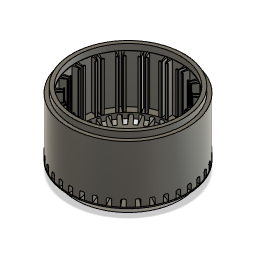
Halbach_Rotor_A (Autodesk Fusion 360 design; units mm, degrees)
Autodesk Fusion 360 part; units mm, degrees
note: some values were not read from the file. Chosen so that the rebuilt part matches the saved one: which face or edge a step refers to.
(part 1 of 3)
sketch "Sketch1" plane through (0, 0, 0) normal (0, 1, 0) x (1, 0, 0)
  line L0 (-5.9762, 42.5827) -> (4.023, 42.711)
  line L1 (-6.5833, 37.3358) -> (-7.4669, 42.3467) construction
  line L2 (-7.4669, 42.3467) -> (-6.3685, 36.1175)
  line L3 (0, 0) -> (7.4669, 42.3467) construction
  arc A0 (-6.7723, 38.4075) -> (-19.5, 33.775) centre (0, 0) ccw construction
  arc A1 (7.4669, 42.3467) -> (-7.4669, 42.3467) centre (0, 0) ccw construction
  line L4 (0, 0) -> (0, 22.1524)
  line L5 (5.4237, 42.6398) -> (7.4669, 42.3467)
  line L6 (4.023, 42.711) -> (4.0904, 37.4578)
  arc A2 (19.5, 33.775) -> (6.7723, 38.4075) centre (0, 0) ccw construction
  line L7 (-7.4669, 42.3467) -> (-5.9762, 42.5827)
  line L8 (-5.9762, 42.5827) -> (-5.912, 37.5831)
  line L9 (5.4238, 42.6403) -> (4.6599, 37.3153)
  line L10 (-5.912, 37.5831) -> (-5.9313, 39.0855)
  line L11 (7.4669, 42.3467) -> (6.4589, 36.6302)
  arc A3 (21.4323, 37.2711) -> (7.4669, 42.3467) centre (0.1099, 0.3541) ccw construction
  arc A4 (-7.2932, 41.3619) -> (-21, 36.3731) centre (0, 0) ccw construction
  line L12 (-5.912, 37.5831) -> (-4.4122, 37.6023)
  line L13 (-4.4122, 37.6023) -> (-4.4057, 37.1024)
  line L14 (-4.4057, 37.1024) -> (-5.9663, 36.8865)
  line L15 (4.0904, 37.4578) -> (2.5905, 37.4386)
  line L16 (2.5905, 37.4386) -> (2.5969, 36.9386)
  line L17 (4.6169, 36.9835) -> (4.6139, 36.9628)
  line L18 (-7.4669, 42.3467) -> (-6.4589, 36.6302)
  line L19 (-9.4242, 41.9378) -> (-7.4669, 42.3467)
  arc A5 (-7.4669, 42.3467) -> (-21.5, 37.2391) centre (0, 0) ccw construction
  line L20 (-23.1994, 36.1854) -> (-21.5, 37.2391)
  arc A6 (-21.5, 37.2391) -> (-32.9399, 27.6399) centre (0, 0) ccw construction
  line L21 (-34.1765, 26.0685) -> (-32.9399, 27.6399)
  arc A7 (-32.9399, 27.6399) -> (-40.4068, 14.7069) centre (0, 0) ccw construction
  line L22 (-41.0313, 12.8073) -> (-40.4068, 14.7069)
  arc A8 (-40.4068, 14.7069) -> (-43, 0) centre (0, 0) ccw construction
  line L23 (-42.9372, -1.9986) -> (-43, 0)
  arc A9 (-43, 0) -> (-40.4068, -14.7069) centre (0, 0) ccw construction
  line L24 (-39.6642, -16.5635) -> (-40.4068, -14.7069)
  arc A10 (-40.4068, -14.7069) -> (-32.9399, -27.6399) centre (0, 0) ccw construction
  line L25 (-31.6071, -29.1305) -> (-32.9399, -27.6399)
  arc A11 (-32.9399, -27.6399) -> (-21.5, -37.2391) centre (0, 0) ccw construction
  line L26 (-19.7377, -38.184) -> (-21.5, -37.2391)
  arc A12 (-21.5, -37.2391) -> (-7.4669, -42.3467) centre (0, 0) ccw construction
  line L27 (-5.4877, -42.6319) -> (-7.4669, -42.3467)
  arc A13 (-7.4669, -42.3467) -> (7.4669, -42.3467) centre (0, 0) ccw construction
  line L28 (21.5, -37.2391) -> (20.1799, -37.9707)
  line L29 (21.5, -37.2391) -> (18.3374, -31.7612)
  line L30 (9.4242, -41.9378) -> (7.4669, -42.3467)
  arc A14 (7.4669, -42.3467) -> (21.5, -37.2391) centre (0, 0) ccw construction
  line L31 (21.5, -37.2391) -> (18.5976, -32.212)
  line L32 (23.1994, -36.1854) -> (21.5, -37.2391)
  arc A15 (21.5, -37.2391) -> (32.9399, -27.6399) centre (0, 0) ccw construction
  line L33 (34.1765, -26.0685) -> (32.9399, -27.6399)
  arc A16 (32.9399, -27.6399) -> (40.4068, -14.7069) centre (0, 0) ccw construction
  line L34 (41.0313, -12.8073) -> (40.4068, -14.7069)
  arc A17 (40.4068, -14.7069) -> (43, 0) centre (0, 0) ccw construction
  line L35 (42.9372, 1.9986) -> (43, 0)
  arc A18 (43, 0) -> (40.4068, 14.7069) centre (0, 0) ccw construction
  line L36 (39.6642, 16.5635) -> (40.4068, 14.7069)
  arc A19 (40.4068, 14.7069) -> (32.9399, 27.6399) centre (0, 0) ccw construction
  line L37 (31.6071, 29.1305) -> (32.9399, 27.6399)
  arc A20 (32.9399, 27.6399) -> (21.5, 37.2391) centre (0, 0) ccw construction
  line L38 (19.7377, 38.184) -> (21.5, 37.2391)
  arc A21 (21.5, 37.2391) -> (7.4669, 42.3467) centre (0, 0) ccw construction
  line L39 (-9.4242, 41.9378) -> (-9.4276, 41.9538)
  arc A22 (-6.5833, 37.3358) -> (-5.9663, 36.8865) centre (-6.0417, 37.4314) ccw
  line L40 (4.73, 37.8039) -> (4.6599, 37.3153)
  line L41 (4.1482, 36.8865) -> (2.5969, 36.9386)
  arc A23 (4.1482, 36.8865) -> (4.6599, 37.3153) centre (4.165, 37.3863) ccw
  line L42 (-18.9559, 32.8326) -> (-21.5, 37.2391) construction
  line L43 (-9.4871, 41.9233) -> (-7.4669, 42.3467)
  line L44 (-8.3107, 36.3322) -> (-8.3064, 36.3118)
  line L45 (-10.8276, 41.5111) -> (-8.9676, 36.5978)
  line L46 (-7.4669, 42.3467) -> (-6.4589, 36.6302)
  line L47 (-9.4872, 41.9238) -> (-8.3837, 36.6587)
  line L48 (-23.1994, 36.1854) -> (-23.208, 36.1993)
  line L49 (-8.4849, 37.1418) -> (-8.3837, 36.6587)
  line L50 (-8.9676, 36.5978) -> (-10.3705, 36.0667)
  line L51 (-20.1799, 37.9707) -> (-18.4097, 33.2945)
  line L52 (-10.3705, 36.0667) -> (-10.1934, 35.5991)
  line L53 (-8.7179, 36.0808) -> (-10.1934, 35.5991)
  line L54 (-16.8298, 33.358) -> (-18.2224, 32.6214)
  line L55 (-21.5, 37.2391) -> (-18.5976, 32.212)
  line L56 (-23.1994, 36.1854) -> (-21.5, 37.2391)
  arc A24 (-7.4669, 42.3467) -> (-21.5, 37.2391) centre (0, 0) ccw construction
  line L57 (-20.1799, 37.9707) -> (-10.8276, 41.5111)
  line L58 (-21.5, 37.2391) -> (-20.1799, 37.9707)
  arc A25 (-18.9559, 32.8326) -> (-18.2224, 32.6214) centre (-18.4796, 33.1076) ccw
  line L59 (-18.4097, 33.2945) -> (-18.9416, 34.6997)
  line L60 (-18.4097, 33.2945) -> (-17.0068, 33.8256)
  line L61 (-17.0068, 33.8256) -> (-16.8298, 33.358)
  line L62 (-21.5, 37.2391) -> (-18.3374, 31.7612)
  arc A26 (-8.7179, 36.0808) -> (-8.3837, 36.6587) centre (-8.873, 36.5561) ccw
  line L63 (-29.0421, 24.3692) -> (-32.9399, 27.6399) construction
  line L64 (-23.2536, 36.1503) -> (-21.5, 37.2391)
  line L65 (-20.2358, 31.2987) -> (-20.2248, 31.2809)
  line L66 (-24.3723, 35.3044) -> (-20.944, 31.3236)
  line L67 (-21.5, 37.2391) -> (-18.5976, 32.212)
  line L68 (-23.2538, 36.1507) -> (-20.4161, 31.5805)
  line L69 (-34.1765, 26.0685) -> (-34.1893, 26.0786)
  line L70 (-20.6765, 31.9999) -> (-20.4161, 31.5805)
  line L71 (-20.944, 31.3236) -> (-22.0806, 30.3448)
  line L72 (-31.9496, 28.7788) -> (-28.6868, 24.9901)
  line L73 (-22.0806, 30.3448) -> (-21.7543, 29.9659)
  line L74 (-20.5325, 30.9232) -> (-21.7543, 29.9659)
  line L75 (-27.2239, 25.5901) -> (-28.2807, 24.4217)
  line L76 (-32.9399, 27.6399) -> (-28.4932, 23.9087)
  line L77 (-34.1765, 26.0685) -> (-32.9399, 27.6399)
  arc A27 (-21.5, 37.2391) -> (-32.9399, 27.6399) centre (0, 0) ccw construction
  line L78 (-31.9496, 28.7788) -> (-24.3723, 35.3044)
  line L79 (-32.9399, 27.6399) -> (-31.9496, 28.7788)
  arc A28 (-29.0421, 24.3692) -> (-28.2807, 24.4217) centre (-28.6886, 24.7906) ccw
  line L80 (-28.6868, 24.9901) -> (-29.6673, 26.1287)
  line L81 (-28.6868, 24.9901) -> (-27.5502, 25.969)
  line L82 (-27.5502, 25.969) -> (-27.2239, 25.5901)
  line L83 (-32.9399, 27.6399) -> (-28.0945, 23.5741)
  arc A29 (-20.5325, 30.9232) -> (-20.4161, 31.5805) centre (-20.8408, 31.3168) ccw
  line L84 (-35.6255, 12.9666) -> (-40.4068, 14.7069) construction
  line L85 (-34.2153, 26.0169) -> (-32.9399, 27.6399)
  line L86 (-29.7202, 22.4901) -> (-29.7038, 22.4772)
  line L87 (-34.9773, 24.8395) -> (-30.3942, 22.2713)
  line L88 (-32.9399, 27.6399) -> (-28.4932, 23.9087)
  line L89 (-34.2157, 26.0173) -> (-29.986, 22.6933)
  line L90 (-41.0313, 12.8073) -> (-41.0468, 12.8124)
  line L91 (-30.3741, 22.9983) -> (-29.986, 22.6933)
  line L92 (-30.3942, 22.2713) -> (-31.1275, 20.9627)
  line L93 (-39.8658, 16.1158) -> (-35.5039, 13.6716)
  line L94 (-31.1275, 20.9627) -> (-30.6913, 20.7183)
  line L95 (-29.8706, 22.0358) -> (-30.6913, 20.7183)
  line L96 (-34.3345, 14.7357) -> (-34.9278, 13.2763)
  line L97 (-40.4068, 14.7069) -> (-34.9521, 12.7215)
  line L98 (-41.0313, 12.8073) -> (-40.4068, 14.7069)
  arc A30 (-32.9399, 27.6399) -> (-40.4068, 14.7069) centre (0, 0) ccw construction
  line L99 (-39.8658, 16.1158) -> (-34.9773, 24.8395)
  line L100 (-40.4068, 14.7069) -> (-39.8658, 16.1158)
  arc A31 (-35.6255, 12.9666) -> (-34.9278, 13.2763) centre (-35.4373, 13.4834) ccw
  line L101 (-35.5039, 13.6716) -> (-36.8147, 14.4061)
  line L102 (-35.5039, 13.6716) -> (-34.7707, 14.9801)
  line L103 (-34.7707, 14.9801) -> (-34.3345, 14.7357)
  line L104 (-40.4068, 14.7069) -> (-34.463, 12.5435)
  arc A32 (-29.8706, 22.0358) -> (-29.986, 22.6933) centre (-30.2949, 22.3001) ccw
  line L105 (-37.9118, 0) -> (-43, 0) construction
  line L106 (-41.0502, 12.7456) -> (-40.4068, 14.7069)
  line L107 (-35.6199, 10.9688) -> (-35.6001, 10.9623)
  line L108 (-41.3635, 11.3786) -> (-36.1784, 10.5327)
  line L109 (-40.4068, 14.7069) -> (-34.9521, 12.7215)
  line L110 (-41.0507, 12.7458) -> (-35.9392, 11.0689)
  line L111 (-42.9372, -1.9986) -> (-42.9535, -1.9991)
  line L112 (-36.4082, 11.2228) -> (-35.9392, 11.0689)
  line L113 (-36.1784, 10.5327) -> (-36.4199, 9.0523)
  line L114 (-42.9735, 1.509) -> (-38.0387, 0.704)
  line L115 (-36.4199, 9.0523) -> (-35.9265, 8.9718)
  line L116 (-35.6058, 10.4905) -> (-35.9265, 8.9718)
  line L117 (-37.3038, 2.1039) -> (-37.3622, 0.5296)
  line L118 (-43, 0) -> (-37.1953, 0)
  line L119 (-42.9372, -1.9986) -> (-43, 0)
  arc A33 (-40.4068, 14.7069) -> (-43, 0) centre (0, 0) ccw construction
  line L120 (-42.9735, 1.509) -> (-41.3635, 11.3786)
  line L121 (-43, 0) -> (-42.9735, 1.509)
  arc A34 (-37.9118, 0) -> (-37.3622, 0.5296) centre (-37.9118, 0.55) ccw
  line L122 (-38.0387, 0.704) -> (-39.5217, 0.9459)
  line L123 (-38.0387, 0.704) -> (-37.7972, 2.1844)
  line L124 (-37.7972, 2.1844) -> (-37.3038, 2.1039)
  line L125 (-43, 0) -> (-36.6747, 0)
  arc A35 (-35.6058, 10.4905) -> (-35.9392, 11.0689) centre (-36.095, 10.5938) ccw
  line L126 (-35.6255, -12.9666) -> (-40.4068, -14.7069) construction
  line L127 (-42.9338, -2.063) -> (-43, 0)
  line L128 (-37.2233, -1.8754) -> (-37.2025, -1.8747)
  line L129 (-42.7607, -3.4548) -> (-37.599, -2.4762)
  line L130 (-43, 0) -> (-37.1953, 0)
  line L131 (-42.9343, -2.0631) -> (-37.5576, -1.8906)
  line L132 (-39.6642, -16.5635) -> (-39.6793, -16.5695)
  line L133 (-38.0509, -1.9064) -> (-37.5576, -1.8906)
  line L134 (-37.599, -2.4762) -> (-37.3196, -3.95)
  line L135 (-40.898, -13.2798) -> (-35.9855, -12.3485)
  line L136 (-37.3196, -3.95) -> (-36.8284, -3.8568)
  line L137 (-37.0465, -2.3201) -> (-36.8284, -3.8568)
  line L138 (-35.7737, -10.7816) -> (-35.2901, -12.281)
  line L139 (-40.4068, -14.7069) -> (-34.9521, -12.7215)
  line L140 (-39.6642, -16.5635) -> (-40.4068, -14.7069)
  arc A36 (-43, 0) -> (-40.4068, -14.7069) centre (0, 0) ccw construction
  line L141 (-40.898, -13.2798) -> (-42.7607, -3.4548)
  line L142 (-40.4068, -14.7069) -> (-40.898, -13.2798)
  arc A37 (-35.6255, -12.9666) -> (-35.2901, -12.281) centre (-35.8136, -12.4498) ccw
  line L143 (-35.9855, -12.3485) -> (-37.4617, -12.6283)
  line L144 (-35.9855, -12.3485) -> (-36.2649, -10.8747)
  line L145 (-36.2649, -10.8747) -> (-35.7737, -10.7816)
  line L146 (-40.4068, -14.7069) -> (-34.463, -12.5435)
  arc A38 (-37.0465, -2.3201) -> (-37.5576, -1.8906) centre (-37.5415, -2.3903) ccw
  line L147 (-29.0421, -24.3692) -> (-32.9399, -27.6399) construction
  line L148 (-39.639, -16.6229) -> (-40.4068, -14.7069)
  line L149 (-34.3371, -14.4934) -> (-34.3177, -14.4857)
  line L150 (-39.0003, -17.8714) -> (-34.4846, -15.1865)
  line L151 (-40.4068, -14.7069) -> (-34.9521, -12.7215)
  line L152 (-39.6395, -16.623) -> (-34.6459, -14.622)
  line L153 (-31.6071, -29.1305) -> (-31.6193, -29.1414)
  line L154 (-35.1041, -14.8056) -> (-34.6459, -14.622)
  line L155 (-34.4846, -15.1865) -> (-33.718, -16.4758)
  line L156 (-33.8896, -26.4669) -> (-29.5919, -23.9115)
  line L157 (-33.718, -16.4758) -> (-33.2882, -16.2203)
  line L158 (-34.0188, -14.8508) -> (-33.2882, -16.2203)
  line L159 (-29.9287, -22.3667) -> (-28.9615, -23.6103)
  line L160 (-32.9399, -27.6399) -> (-28.4932, -23.9087)
  line L161 (-31.6071, -29.1305) -> (-32.9399, -27.6399)
  arc A39 (-40.4068, -14.7069) -> (-32.9399, -27.6399) centre (0, 0) ccw construction
  line L162 (-33.8896, -26.4669) -> (-39.0003, -17.8714)
  line L163 (-32.9399, -27.6399) -> (-33.8896, -26.4669)
  arc A40 (-29.0421, -24.3692) -> (-28.9615, -23.6103) centre (-29.3957, -23.9479) ccw
  line L164 (-29.5919, -23.9115) -> (-30.8834, -24.6794)
  line L165 (-29.5919, -23.9115) -> (-30.3585, -22.6222)
  line L166 (-30.3585, -22.6222) -> (-29.9287, -22.3667)
  line L167 (-32.9399, -27.6399) -> (-28.0945, -23.5741)
  arc A41 (-34.0188, -14.8508) -> (-34.6459, -14.622) centre (-34.46, -15.0861) ccw
  line L168 (-18.9559, -32.8326) -> (-21.5, -37.2391) construction
  line L169 (-31.5631, -29.1777) -> (-32.9399, -27.6399)
  line L170 (-27.3092, -25.3633) -> (-27.2937, -25.3494)
  line L171 (-30.5359, -30.1325) -> (-27.2108, -26.0651)
  line L172 (-32.9399, -27.6399) -> (-28.4932, -23.9087)
  line L173 (-31.5635, -29.178) -> (-27.5555, -25.5898)
  line L174 (-19.7377, -38.184) -> (-19.7455, -38.1984)
  line L175 (-27.9233, -25.9191) -> (-27.5555, -25.5898)
  line L176 (-27.2108, -26.0651) -> (-26.0495, -27.0145)
  line L177 (-22.7936, -36.4616) -> (-19.6291, -32.5905)
  line L178 (-26.0495, -27.0145) -> (-25.733, -26.6273)
  line L179 (-26.888, -25.5903) -> (-25.733, -26.6273)
  line L180 (-20.474, -31.254) -> (-19.1397, -32.0918)
  line L181 (-21.5, -37.2391) -> (-18.5976, -32.212)
  line L182 (-19.7377, -38.184) -> (-21.5, -37.2391)
  arc A42 (-32.9399, -27.6399) -> (-21.5, -37.2391) centre (0, 0) ccw construction
  line L183 (-22.7936, -36.4616) -> (-30.5359, -30.1325)
  line L184 (-21.5, -37.2391) -> (-22.7936, -36.4616)
  arc A43 (-18.9559, -32.8326) -> (-19.1397, -32.0918) centre (-19.4322, -32.5576) ccw
  line L185 (-19.6291, -32.5905) -> (-20.58, -33.7538)
  line L186 (-19.6291, -32.5905) -> (-20.7904, -31.6411)
  line L187 (-20.7904, -31.6411) -> (-20.474, -31.254)
  line L188 (-21.5, -37.2391) -> (-18.3374, -31.7612)
  arc A44 (-26.888, -25.5903) -> (-27.5555, -25.5898) centre (-27.222, -25.9623) ccw
  line L189 (-6.5833, -37.3358) -> (-7.4669, -42.3467) construction
  line L190 (-19.6803, -38.2133) -> (-21.5, -37.2391)
  line L191 (-16.9875, -33.1741) -> (-16.9777, -33.1557)
  line L192 (-18.3884, -38.7592) -> (-16.655, -33.7998)
  line L193 (-21.5, -37.2391) -> (-18.5976, -32.212)
  line L194 (-19.6805, -38.2137) -> (-17.1415, -33.4711)
  line L195 (-5.4877, -42.6319) -> (-5.49, -42.6481)
  line L196 (-17.3745, -33.9063) -> (-17.1415, -33.4711)
  line L197 (-16.655, -33.7998) -> (-15.239, -34.2947)
  line L198 (-8.9484, -42.0586) -> (-7.2987, -37.3386)
  line L199 (-15.239, -34.2947) -> (-15.0741, -33.8227)
  line L200 (-16.514, -33.2432) -> (-15.0741, -33.8227)
  line L201 (-8.5497, -36.3717) -> (-7.0094, -36.7026)
  line L202 (-7.4669, -42.3467) -> (-6.4589, -36.6302)
  line L203 (-5.4877, -42.6319) -> (-7.4669, -42.3467)
  arc A45 (-21.5, -37.2391) -> (-7.4669, -42.3467) centre (0, 0) ccw construction
  line L204 (-8.9484, -42.0586) -> (-18.3884, -38.7592)
  line L205 (-7.4669, -42.3467) -> (-8.9484, -42.0586)
  arc A46 (-6.5833, -37.3358) -> (-7.0094, -36.7026) centre (-7.125, -37.2403) ccw
  line L206 (-7.2987, -37.3386) -> (-7.7944, -38.757)
  line L207 (-7.2987, -37.3386) -> (-8.7147, -36.8437)
  line L208 (-8.7147, -36.8437) -> (-8.5497, -36.3717)
  line L209 (-7.4669, -42.3467) -> (-6.3685, -36.1175)
  arc A47 (-16.514, -33.2432) -> (-17.1415, -33.4711) centre (-16.7007, -33.7071) ccw
  line L210 (6.5833, -37.3358) -> (7.4669, -42.3467) construction
  line L211 (-5.4237, -42.6398) -> (-7.4669, -42.3467)
  line L212 (-4.6169, -36.9835) -> (-4.6139, -36.9628)
  line L213 (-4.023, -42.711) -> (-4.0904, -37.4578)
  line L214 (-7.4669, -42.3467) -> (-6.4589, -36.6302)
  line L215 (-5.4238, -42.6403) -> (-4.6599, -37.3153)
  line L216 (9.4242, -41.9378) -> (9.4276, -41.9538)
  line L217 (-4.73, -37.8039) -> (-4.6599, -37.3153)
  line L218 (-4.0904, -37.4578) -> (-2.5905, -37.4386)
  line L219 (5.9762, -42.5827) -> (5.912, -37.5831)
  line L220 (-2.5905, -37.4386) -> (-2.5969, -36.9386)
  line L221 (-4.1482, -36.8865) -> (-2.5969, -36.9386)
  line L222 (4.4057, -37.1024) -> (5.9663, -36.8865)
  line L223 (7.4669, -42.3467) -> (6.4589, -36.6302)
  line L224 (9.4242, -41.9378) -> (7.4669, -42.3467)
  arc A48 (-7.4669, -42.3467) -> (7.4669, -42.3467) centre (0, 0) ccw construction
  line L225 (5.9762, -42.5827) -> (-4.023, -42.711)
  line L226 (7.4669, -42.3467) -> (5.9762, -42.5827)
  arc A49 (6.5833, -37.3358) -> (5.9663, -36.8865) centre (6.0417, -37.4314) ccw
  line L227 (5.912, -37.5831) -> (5.9313, -39.0855)
  line L228 (5.912, -37.5831) -> (4.4122, -37.6023)
  line L229 (4.4122, -37.6023) -> (4.4057, -37.1024)
  line L230 (7.4669, -42.3467) -> (6.3685, -36.1175)
  arc A50 (-4.1482, -36.8865) -> (-4.6599, -37.3153) centre (-4.165, -37.3863) ccw
  line L231 (18.9559, -32.8326) -> (21.5, -37.2391) construction
  line L232 (9.4871, -41.9233) -> (7.4669, -42.3467)
  line L233 (8.3107, -36.3322) -> (8.3064, -36.3118)
  line L234 (10.8276, -41.5111) -> (8.9676, -36.5978)
  line L235 (7.4669, -42.3467) -> (6.4589, -36.6302)
  line L236 (9.4872, -41.9238) -> (8.3837, -36.6587)
  line L237 (23.1994, -36.1854) -> (23.208, -36.1993)
  line L238 (8.4849, -37.1418) -> (8.3837, -36.6587)
  line L239 (8.9676, -36.5978) -> (10.3705, -36.0667)
  line L240 (20.1799, -37.9707) -> (18.4097, -33.2945)
  line L241 (10.3705, -36.0667) -> (10.1934, -35.5991)
  line L242 (8.7179, -36.0808) -> (10.1934, -35.5991)
  line L243 (16.8298, -33.358) -> (18.2224, -32.6214)
  line L244 (21.5, -37.2391) -> (18.5976, -32.212)
  line L245 (23.1994, -36.1854) -> (21.5, -37.2391)
  arc A51 (7.4669, -42.3467) -> (21.5, -37.2391) centre (0, 0) ccw construction
  line L246 (20.1799, -37.9707) -> (10.8276, -41.5111)
  line L247 (21.5, -37.2391) -> (20.1799, -37.9707)
  arc A52 (18.9559, -32.8326) -> (18.2224, -32.6214) centre (18.4796, -33.1076) ccw
  line L248 (18.4097, -33.2945) -> (18.9416, -34.6997)
  line L249 (18.4097, -33.2945) -> (17.0068, -33.8256)
  line L250 (17.0068, -33.8256) -> (16.8298, -33.358)
  line L251 (21.5, -37.2391) -> (18.3374, -31.7612)
  arc A53 (8.7179, -36.0808) -> (8.3837, -36.6587) centre (8.873, -36.5561) ccw
  line L252 (29.0421, -24.3692) -> (32.9399, -27.6399) construction
  line L253 (23.2536, -36.1503) -> (21.5, -37.2391)
  line L254 (20.2358, -31.2987) -> (20.2248, -31.2809)
  line L255 (24.3723, -35.3044) -> (20.944, -31.3236)
  line L256 (21.5, -37.2391) -> (18.5976, -32.212)
  line L257 (23.2538, -36.1507) -> (20.4161, -31.5805)
  line L258 (34.1765, -26.0685) -> (34.1893, -26.0786)
  line L259 (20.6765, -31.9999) -> (20.4161, -31.5805)
  line L260 (20.944, -31.3236) -> (22.0806, -30.3448)
  line L261 (31.9496, -28.7788) -> (28.6868, -24.9901)
  line L262 (22.0806, -30.3448) -> (21.7543, -29.9659)
  line L263 (20.5325, -30.9232) -> (21.7543, -29.9659)
  line L264 (27.2239, -25.5901) -> (28.2807, -24.4217)
  line L265 (32.9399, -27.6399) -> (28.4932, -23.9087)
  line L266 (34.1765, -26.0685) -> (32.9399, -27.6399)
  arc A54 (21.5, -37.2391) -> (32.9399, -27.6399) centre (0, 0) ccw construction
  line L267 (31.9496, -28.7788) -> (24.3723, -35.3044)
  line L268 (32.9399, -27.6399) -> (31.9496, -28.7788)
  arc A55 (29.0421, -24.3692) -> (28.2807, -24.4217) centre (28.6886, -24.7906) ccw
  line L269 (28.6868, -24.9901) -> (29.6673, -26.1287)
  line L270 (28.6868, -24.9901) -> (27.5502, -25.969)
  line L271 (27.5502, -25.969) -> (27.2239, -25.5901)
  line L272 (32.9399, -27.6399) -> (28.0945, -23.5741)
  arc A56 (20.5325, -30.9232) -> (20.4161, -31.5805) centre (20.8408, -31.3168) ccw
  line L273 (35.6255, -12.9666) -> (40.4068, -14.7069) construction
  line L274 (34.2153, -26.0169) -> (32.9399, -27.6399)
  line L275 (29.7202, -22.4901) -> (29.7038, -22.4772)
  line L276 (34.9773, -24.8395) -> (30.3942, -22.2713)
  line L277 (32.9399, -27.6399) -> (28.4932, -23.9087)
  line L278 (34.2157, -26.0173) -> (29.986, -22.6933)
  line L279 (41.0313, -12.8073) -> (41.0468, -12.8124)
  line L280 (30.3741, -22.9983) -> (29.986, -22.6933)
  line L281 (30.3942, -22.2713) -> (31.1275, -20.9627)
  line L282 (39.8658, -16.1158) -> (35.5039, -13.6716)
  line L283 (31.1275, -20.9627) -> (30.6913, -20.7183)
  line L284 (29.8706, -22.0358) -> (30.6913, -20.7183)
  line L285 (34.3345, -14.7357) -> (34.9278, -13.2763)
  line L286 (40.4068, -14.7069) -> (34.9521, -12.7215)
  line L287 (41.0313, -12.8073) -> (40.4068, -14.7069)
  arc A57 (32.9399, -27.6399) -> (40.4068, -14.7069) centre (0, 0) ccw construction
  line L288 (39.8658, -16.1158) -> (34.9773, -24.8395)
  line L289 (40.4068, -14.7069) -> (39.8658, -16.1158)
  arc A58 (35.6255, -12.9666) -> (34.9278, -13.2763) centre (35.4373, -13.4834) ccw
  line L290 (35.5039, -13.6716) -> (36.8147, -14.4061)
  line L291 (35.5039, -13.6716) -> (34.7707, -14.9801)
  line L292 (34.7707, -14.9801) -> (34.3345, -14.7357)
  line L293 (40.4068, -14.7069) -> (34.463, -12.5435)
  arc A59 (29.8706, -22.0358) -> (29.986, -22.6933) centre (30.2949, -22.3001) ccw
  line L294 (37.9118, 0) -> (43, 0) construction
  line L295 (41.0502, -12.7456) -> (40.4068, -14.7069)
  line L296 (35.6199, -10.9688) -> (35.6001, -10.9623)
  line L297 (41.3635, -11.3786) -> (36.1784, -10.5327)
  line L298 (40.4068, -14.7069) -> (34.9521, -12.7215)
  line L299 (41.0507, -12.7458) -> (35.9392, -11.0689)
  line L300 (42.9372, 1.9986) -> (42.9535, 1.9991)
  line L301 (36.4082, -11.2228) -> (35.9392, -11.0689)
  line L302 (36.1784, -10.5327) -> (36.4199, -9.0523)
  line L303 (42.9735, -1.509) -> (38.0387, -0.704)
  line L304 (36.4199, -9.0523) -> (35.9265, -8.9718)
  line L305 (35.6058, -10.4905) -> (35.9265, -8.9718)
  line L306 (37.3038, -2.1039) -> (37.3622, -0.5296)
  line L307 (43, 0) -> (37.1953, 0)
  line L308 (42.9372, 1.9986) -> (43, 0)
  arc A60 (40.4068, -14.7069) -> (43, 0) centre (0, 0) ccw construction
  line L309 (42.9735, -1.509) -> (41.3635, -11.3786)
  line L310 (43, 0) -> (42.9735, -1.509)
  arc A61 (37.9118, 0) -> (37.3622, -0.5296) centre (37.9118, -0.55) ccw
  line L311 (38.0387, -0.704) -> (39.5217, -0.9459)
  line L312 (38.0387, -0.704) -> (37.7972, -2.1844)
  line L313 (37.7972, -2.1844) -> (37.3038, -2.1039)
  line L314 (43, 0) -> (36.6747, 0)
  arc A62 (35.6058, -10.4905) -> (35.9392, -11.0689) centre (36.095, -10.5938) ccw
  line L315 (35.6255, 12.9666) -> (40.4068, 14.7069) construction
  line L316 (42.9338, 2.063) -> (43, 0)
  line L317 (37.2233, 1.8754) -> (37.2025, 1.8747)
  line L318 (42.7607, 3.4548) -> (37.599, 2.4762)
  line L319 (43, 0) -> (37.1953, 0)
  line L320 (42.9343, 2.0631) -> (37.5576, 1.8906)
  line L321 (39.6642, 16.5635) -> (39.6793, 16.5695)
  line L322 (38.0509, 1.9064) -> (37.5576, 1.8906)
  line L323 (37.599, 2.4762) -> (37.3196, 3.95)
  line L324 (40.898, 13.2798) -> (35.9855, 12.3485)
  line L325 (37.3196, 3.95) -> (36.8284, 3.8568)
  line L326 (37.0465, 2.3201) -> (36.8284, 3.8568)
  line L327 (35.7737, 10.7816) -> (35.2901, 12.281)
  line L328 (40.4068, 14.7069) -> (34.9521, 12.7215)
  line L329 (39.6642, 16.5635) -> (40.4068, 14.7069)
  arc A63 (43, 0) -> (40.4068, 14.7069) centre (0, 0) ccw construction
  line L330 (40.898, 13.2798) -> (42.7607, 3.4548)
  line L331 (40.4068, 14.7069) -> (40.898, 13.2798)
  arc A64 (35.6255, 12.9666) -> (35.2901, 12.281) centre (35.8136, 12.4498) ccw
  line L332 (35.9855, 12.3485) -> (37.4617, 12.6283)
  line L333 (35.9855, 12.3485) -> (36.2649, 10.8747)
  line L334 (36.2649, 10.8747) -> (35.7737, 10.7816)
  line L335 (40.4068, 14.7069) -> (34.463, 12.5435)
  arc A65 (37.0465, 2.3201) -> (37.5576, 1.8906) centre (37.5415, 2.3903) ccw
  line L336 (29.0421, 24.3692) -> (32.9399, 27.6399) construction
  line L337 (39.639, 16.6229) -> (40.4068, 14.7069)
  line L338 (34.3371, 14.4934) -> (34.3177, 14.4857)
  line L339 (39.0003, 17.8714) -> (34.4846, 15.1865)
  line L340 (40.4068, 14.7069) -> (34.9521, 12.7215)
  line L341 (39.6395, 16.623) -> (34.6459, 14.622)
  line L342 (31.6071, 29.1305) -> (31.6193, 29.1414)
  line L343 (35.1041, 14.8056) -> (34.6459, 14.622)
  line L344 (34.4846, 15.1865) -> (33.718, 16.4758)
  line L345 (33.8896, 26.4669) -> (29.5919, 23.9115)
  line L346 (33.718, 16.4758) -> (33.2882, 16.2203)
  line L347 (34.0188, 14.8508) -> (33.2882, 16.2203)
  line L348 (29.9287, 22.3667) -> (28.9615, 23.6103)
  line L349 (32.9399, 27.6399) -> (28.4932, 23.9087)
  line L350 (31.6071, 29.1305) -> (32.9399, 27.6399)
  arc A66 (40.4068, 14.7069) -> (32.9399, 27.6399) centre (0, 0) ccw construction
  line L351 (33.8896, 26.4669) -> (39.0003, 17.8714)
  line L352 (32.9399, 27.6399) -> (33.8896, 26.4669)
  arc A67 (29.0421, 24.3692) -> (28.9615, 23.6103) centre (29.3957, 23.9479) ccw
  line L353 (29.5919, 23.9115) -> (30.8834, 24.6794)
  line L354 (29.5919, 23.9115) -> (30.3585, 22.6222)
  line L355 (30.3585, 22.6222) -> (29.9287, 22.3667)
  line L356 (32.9399, 27.6399) -> (28.0945, 23.5741)
  arc A68 (34.0188, 14.8508) -> (34.6459, 14.622) centre (34.46, 15.0861) ccw
  line L357 (18.9559, 32.8326) -> (21.5, 37.2391) construction
  line L358 (31.5631, 29.1777) -> (32.9399, 27.6399)
  line L359 (27.3092, 25.3633) -> (27.2937, 25.3494)
  line L360 (30.5359, 30.1325) -> (27.2108, 26.0651)
  line L361 (32.9399, 27.6399) -> (28.4932, 23.9087)
  line L362 (31.5635, 29.178) -> (27.5555, 25.5898)
  line L363 (19.7377, 38.184) -> (19.7455, 38.1984)
  line L364 (27.9233, 25.9191) -> (27.5555, 25.5898)
  line L365 (27.2108, 26.0651) -> (26.0495, 27.0145)
  line L366 (22.7936, 36.4616) -> (19.6291, 32.5905)
  line L367 (26.0495, 27.0145) -> (25.733, 26.6273)
  line L368 (26.888, 25.5903) -> (25.733, 26.6273)
  line L369 (20.474, 31.254) -> (19.1397, 32.0918)
  line L370 (21.5, 37.2391) -> (18.5976, 32.212)
  line L371 (19.7377, 38.184) -> (21.5, 37.2391)
  arc A69 (32.9399, 27.6399) -> (21.5, 37.2391) centre (0, 0) ccw construction
  line L372 (22.7936, 36.4616) -> (30.5359, 30.1325)
  line L373 (21.5, 37.2391) -> (22.7936, 36.4616)
  arc A70 (18.9559, 32.8326) -> (19.1397, 32.0918) centre (19.4322, 32.5576) ccw
  line L374 (19.6291, 32.5905) -> (20.58, 33.7538)
  line L375 (19.6291, 32.5905) -> (20.7904, 31.6411)
  line L376 (20.7904, 31.6411) -> (20.474, 31.254)
  line L377 (21.5, 37.2391) -> (18.3374, 31.7612)
  arc A71 (26.888, 25.5903) -> (27.5555, 25.5898) centre (27.222, 25.9623) ccw
  line L378 (6.5833, 37.3358) -> (7.4669, 42.3467) construction
  line L379 (19.6803, 38.2133) -> (21.5, 37.2391)
  line L380 (16.9875, 33.1741) -> (16.9777, 33.1557)
  line L381 (18.3884, 38.7592) -> (16.655, 33.7998)
  line L382 (21.5, 37.2391) -> (18.5976, 32.212)
  line L383 (19.6805, 38.2137) -> (17.1415, 33.4711)
  line L384 (5.4877, 42.6319) -> (5.49, 42.6481)
  line L385 (17.3745, 33.9063) -> (17.1415, 33.4711)
  line L386 (16.655, 33.7998) -> (15.239, 34.2947)
  line L387 (8.9484, 42.0586) -> (7.2987, 37.3386)
  line L388 (15.239, 34.2947) -> (15.0741, 33.8227)
  line L389 (16.514, 33.2432) -> (15.0741, 33.8227)
  line L390 (8.5497, 36.3717) -> (7.0094, 36.7026)
  line L391 (7.4669, 42.3467) -> (6.4589, 36.6302)
  line L392 (5.4877, 42.6319) -> (7.4669, 42.3467)
  arc A72 (21.5, 37.2391) -> (7.4669, 42.3467) centre (0, 0) ccw construction
  line L393 (8.9484, 42.0586) -> (18.3884, 38.7592)
  line L394 (7.4669, 42.3467) -> (8.9484, 42.0586)
  arc A73 (6.5833, 37.3358) -> (7.0094, 36.7026) centre (7.125, 37.2403) ccw
  line L395 (7.2987, 37.3386) -> (7.7944, 38.757)
  line L396 (7.2987, 37.3386) -> (8.7147, 36.8437)
  line L397 (8.7147, 36.8437) -> (8.5497, 36.3717)
  line L398 (7.4669, 42.3467) -> (6.3685, 36.1175)
  arc A74 (16.514, 33.2432) -> (17.1415, 33.4711) centre (16.7007, 33.7071) ccw
  circle A75 centre (0, 0) radius 49
  line L399 (-5.9663, 36.8865) -> (5.7522, 36.8865)
  point P0 (4.0904, 37.4578)
  point P1 (16.3645, 32.9385)
  point P2 (19.5, 33.775)
  point P3 (6.7723, 38.4075)
  point P4 (-8.6365, 35.7513)
  point P5 (-7.2932, 41.3619)
  point P6 (-6.7723, 38.4075)
  point P7 (-19.5, 33.775)
  point P8 (-19.5, 33.775)
  point P9 (-6.7723, 38.4075)
  point P10 (-8.9676, 36.5978)
  point P11 (-19.5, 33.775)
  point P12 (-21, 36.3731)
  point P13 (-21, 36.3731)
  point P14 (-20.3434, 30.6413)
  point P15 (-7.4669, 42.3467)
  point P16 (-6.7723, 38.4075)
  point P17 (-29.8757, 25.0687)
  point P18 (-19.5, 33.775)
  point P19 (-20.944, 31.3236)
  point P20 (-29.8757, 25.0687)
  point P21 (-32.1739, 26.9971)
  point P22 (-32.1739, 26.9971)
  point P23 (-29.5965, 21.8356)
  point P24 (-21.5, 37.2391)
  point P25 (-19.5, 33.775)
  point P26 (-36.648, 13.3388)
  point P27 (-29.8757, 25.0687)
  point P28 (-30.3942, 22.2713)
  point P29 (-36.648, 13.3388)
  point P30 (-39.4671, 14.3648)
  point P31 (-39.4671, 14.3648)
  point P32 (-35.2798, 10.3962)
  point P33 (-32.9399, 27.6399)
  point P34 (-29.8757, 25.0687)
  point P35 (-39, 0)
  point P36 (-36.648, 13.3388)
  point P37 (-36.1784, 10.5327)
  point P38 (-39, 0)
  point P39 (-42, 0)
  point P40 (-42, 0)
  point P41 (-36.7079, -2.2972)
  point P42 (-40.4068, 14.7069)
  point P43 (-36.648, 13.3388)
  point P44 (-36.648, -13.3388)
  point P45 (-39, 0)
  point P46 (-37.599, -2.4762)
  point P47 (-36.648, -13.3388)
  point P48 (-39.4671, -14.3648)
  point P49 (-39.4671, -14.3648)
  point P50 (-33.7084, -14.7135)
  point P51 (-43, 0)
  point P52 (-39, 0)
  point P53 (-29.8757, -25.0687)
  point P54 (-36.648, -13.3388)
  point P55 (-34.4846, -15.1865)
  point P56 (-29.8757, -25.0687)
  point P57 (-32.1739, -26.9971)
  point P58 (-32.1739, -26.9971)
  point P59 (-26.6432, -25.3551)
  point P60 (-40.4068, -14.7069)
  point P61 (-36.648, -13.3388)
  point P62 (-19.5, -33.775)
  point P63 (-29.8757, -25.0687)
  point P64 (-27.2108, -26.0651)
  point P65 (-19.5, -33.775)
  point P66 (-21, -36.3731)
  point P67 (-21, -36.3731)
  point P68 (-16.3645, -32.9385)
  point P69 (-32.9399, -27.6399)
  point P70 (-29.8757, -25.0687)
  point P71 (-6.7723, -38.4075)
  point P72 (-19.5, -33.775)
  point P73 (-16.655, -33.7998)
  point P74 (-6.7723, -38.4075)
  point P75 (-7.2932, -41.3619)
  point P76 (-7.2932, -41.3619)
  point P77 (-4.112, -36.5491)
  point P78 (-21.5, -37.2391)
  point P79 (-19.5, -33.775)
  point P80 (6.7723, -38.4075)
  point P81 (-6.7723, -38.4075)
  point P82 (-4.0904, -37.4578)
  point P83 (6.7723, -38.4075)
  point P84 (7.2932, -41.3619)
  point P85 (7.2932, -41.3619)
  point P86 (8.6365, -35.7513)
  point P87 (-7.4669, -42.3467)
  point P88 (-6.7723, -38.4075)
  point P89 (19.5, -33.775)
  point P90 (6.7723, -38.4075)
  point P91 (8.9676, -36.5978)
  point P92 (19.5, -33.775)
  point P93 (21, -36.3731)
  point P94 (21, -36.3731)
  point P95 (20.3434, -30.6413)
  point P96 (7.4669, -42.3467)
  point P97 (6.7723, -38.4075)
  point P98 (29.8757, -25.0687)
  point P99 (19.5, -33.775)
  point P100 (20.944, -31.3236)
  point P101 (29.8757, -25.0687)
  point P102 (32.1739, -26.9971)
  point P103 (32.1739, -26.9971)
  point P104 (29.5965, -21.8356)
  point P105 (21.5, -37.2391)
  point P106 (19.5, -33.775)
  point P107 (36.648, -13.3388)
  point P108 (29.8757, -25.0687)
  point P109 (30.3942, -22.2713)
  point P110 (36.648, -13.3388)
  point P111 (39.4671, -14.3648)
  point P112 (39.4671, -14.3648)
  point P113 (35.2798, -10.3962)
  point P114 (32.9399, -27.6399)
  point P115 (29.8757, -25.0687)
  point P116 (39, 0)
  point P117 (36.648, -13.3388)
  point P118 (36.1784, -10.5327)
  point P119 (39, 0)
  point P120 (42, 0)
  point P121 (42, 0)
  point P122 (36.7079, 2.2972)
  point P123 (40.4068, -14.7069)
  point P124 (36.648, -13.3388)
  point P125 (36.648, 13.3388)
  point P126 (39, 0)
  point P127 (37.599, 2.4762)
  point P128 (36.648, 13.3388)
  point P129 (39.4671, 14.3648)
  point P130 (39.4671, 14.3648)
  point P131 (33.7084, 14.7135)
  point P132 (43, 0)
  point P133 (39, 0)
  point P134 (29.8757, 25.0687)
  point P135 (36.648, 13.3388)
  point P136 (34.4846, 15.1865)
  point P137 (29.8757, 25.0687)
  point P138 (32.1739, 26.9971)
  point P139 (32.1739, 26.9971)
  point P140 (26.6432, 25.3551)
  point P141 (40.4068, 14.7069)
  point P142 (36.648, 13.3388)
  point P143 (19.5, 33.775)
  point P144 (29.8757, 25.0687)
  point P145 (27.2108, 26.0651)
  point P146 (19.5, 33.775)
  point P147 (21, 36.3731)
  point P148 (21, 36.3731)
  point P149 (16.3645, 32.9385)
  point P150 (32.9399, 27.6399)
  point P151 (29.8757, 25.0687)
  point P152 (6.7723, 38.4075)
  point P153 (19.5, 33.775)
  point P154 (16.655, 33.7998)
  point P155 (6.7723, 38.4075)
  point P156 (7.2932, 41.3619)
  point P157 (7.2932, 41.3619)
  point P158 (21.5, 37.2391)
  point P159 (19.5, 33.775)
  point P160 (-6.7723, 38.4075)
  point P161 (-21, 36.3731)
  point P162 (-21.5, 37.2391)
  point P163 (-7.4669, 42.3467)
  point P164 (-20.944, 31.3236)
  point P165 (-19.5, 33.775)
  point P166 (-6.7723, 38.4075)
  point P167 (-6.7723, 38.4075)
  point P168 (-7.2932, 41.3619)
  point P169 (-20.3434, 30.6413)
  point P170 (-7.2932, 41.3619)
  point P171 (-7.4669, 42.3467)
  point P172 (-8.9676, 36.5978)
  point P173 (-19.5, 33.775)
  point P174 (-21.5, 37.2391)
  point P175 (-19.5, 33.775)
  point P176 (-19.5, 33.775)
  point P177 (-21, 36.3731)
  point P178 (-6.7723, 38.4075)
  point P179 (-19.5, 33.775)
  point P180 (-32.1739, 26.9971)
  point P181 (-32.9399, 27.6399)
  point P182 (-21.5, 37.2391)
  point P183 (-30.3942, 22.2713)
  point P184 (-29.8757, 25.0687)
  point P185 (-19.5, 33.775)
  point P186 (-19.5, 33.775)
  point P187 (-21, 36.3731)
  point P188 (-29.5965, 21.8356)
  point P189 (-21, 36.3731)
  point P190 (-21.5, 37.2391)
  point P191 (-20.944, 31.3236)
  point P192 (-29.8757, 25.0687)
  point P193 (-32.9399, 27.6399)
  point P194 (-29.8757, 25.0687)
  point P195 (-29.8757, 25.0687)
  point P196 (-32.1739, 26.9971)
  point P197 (-19.5, 33.775)
  point P198 (-29.8757, 25.0687)
  point P199 (-39.4671, 14.3648)
  point P200 (-40.4068, 14.7069)
  point P201 (-32.9399, 27.6399)
  point P202 (-36.1784, 10.5327)
  point P203 (-36.648, 13.3388)
  point P204 (-29.8757, 25.0687)
  point P205 (-29.8757, 25.0687)
  point P206 (-32.1739, 26.9971)
  point P207 (-35.2798, 10.3962)
  point P208 (-32.1739, 26.9971)
  point P209 (-32.9399, 27.6399)
  point P210 (-30.3942, 22.2713)
  point P211 (-36.648, 13.3388)
  point P212 (-40.4068, 14.7069)
  point P213 (-36.648, 13.3388)
  point P214 (-36.648, 13.3388)
  point P215 (-39.4671, 14.3648)
  point P216 (-29.8757, 25.0687)
  point P217 (-36.648, 13.3388)
  point P218 (-42, 0)
  point P219 (-43, 0)
  point P220 (-40.4068, 14.7069)
  point P221 (-37.599, -2.4762)
  point P222 (-39, 0)
  point P223 (-36.648, 13.3388)
  point P224 (-36.648, 13.3388)
  point P225 (-39.4671, 14.3648)
  point P226 (-36.7079, -2.2972)
  point P227 (-39.4671, 14.3648)
  point P228 (-40.4068, 14.7069)
  point P229 (-36.1784, 10.5327)
  point P230 (-39, 0)
  point P231 (-43, 0)
  point P232 (-39, 0)
  point P233 (-39, 0)
  point P234 (-42, 0)
  point P235 (-36.648, 13.3388)
  point P236 (-39, 0)
  point P237 (-39.4671, -14.3648)
  point P238 (-40.4068, -14.7069)
  point P239 (-43, 0)
  point P240 (-34.4846, -15.1865)
  point P241 (-36.648, -13.3388)
  point P242 (-39, 0)
  point P243 (-39, 0)
  point P244 (-42, 0)
  point P245 (-33.7084, -14.7135)
  point P246 (-42, 0)
  point P247 (-43, 0)
  point P248 (-37.599, -2.4762)
  point P249 (-36.648, -13.3388)
  point P250 (-40.4068, -14.7069)
  point P251 (-36.648, -13.3388)
  point P252 (-36.648, -13.3388)
  point P253 (-39.4671, -14.3648)
  point P254 (-39, 0)
  point P255 (-36.648, -13.3388)
  point P256 (-32.1739, -26.9971)
  point P257 (-32.9399, -27.6399)
  point P258 (-40.4068, -14.7069)
  point P259 (-27.2108, -26.0651)
  point P260 (-29.8757, -25.0687)
  point P261 (-36.648, -13.3388)
  point P262 (-36.648, -13.3388)
  point P263 (-39.4671, -14.3648)
  point P264 (-26.6432, -25.3551)
  point P265 (-39.4671, -14.3648)
  point P266 (-40.4068, -14.7069)
  point P267 (-34.4846, -15.1865)
  point P268 (-29.8757, -25.0687)
  point P269 (-32.9399, -27.6399)
  point P270 (-29.8757, -25.0687)
  point P271 (-29.8757, -25.0687)
  point P272 (-32.1739, -26.9971)
  point P273 (-36.648, -13.3388)
  point P274 (-29.8757, -25.0687)
  point P275 (-21, -36.3731)
  point P276 (-21.5, -37.2391)
  point P277 (-32.9399, -27.6399)
  point P278 (-16.655, -33.7998)
  point P279 (-19.5, -33.775)
  point P280 (-29.8757, -25.0687)
  point P281 (-29.8757, -25.0687)
  point P282 (-32.1739, -26.9971)
  point P283 (-16.3645, -32.9385)
  point P284 (-32.1739, -26.9971)
  point P285 (-32.9399, -27.6399)
  point P286 (-27.2108, -26.0651)
  point P287 (-19.5, -33.775)
  point P288 (-21.5, -37.2391)
  point P289 (-19.5, -33.775)
  point P290 (-19.5, -33.775)
  point P291 (-21, -36.3731)
  point P292 (-29.8757, -25.0687)
  point P293 (-19.5, -33.775)
  point P294 (-7.2932, -41.3619)
  point P295 (-7.4669, -42.3467)
  point P296 (-21.5, -37.2391)
  point P297 (-4.0904, -37.4578)
  point P298 (-6.7723, -38.4075)
  point P299 (-19.5, -33.775)
  point P300 (-19.5, -33.775)
  point P301 (-21, -36.3731)
  point P302 (-4.112, -36.5491)
  point P303 (-21, -36.3731)
  point P304 (-21.5, -37.2391)
  point P305 (-16.655, -33.7998)
  point P306 (-6.7723, -38.4075)
  point P307 (-7.4669, -42.3467)
  point P308 (-6.7723, -38.4075)
  point P309 (-6.7723, -38.4075)
  point P310 (-7.2932, -41.3619)
  point P311 (-19.5, -33.775)
  point P312 (-6.7723, -38.4075)
  point P313 (7.2932, -41.3619)
  point P314 (7.4669, -42.3467)
  point P315 (-7.4669, -42.3467)
  point P316 (8.9676, -36.5978)
  point P317 (6.7723, -38.4075)
  point P318 (-6.7723, -38.4075)
  point P319 (-6.7723, -38.4075)
  point P320 (-7.2932, -41.3619)
  point P321 (8.6365, -35.7513)
  point P322 (-7.2932, -41.3619)
  point P323 (-7.4669, -42.3467)
  point P324 (-4.0904, -37.4578)
  point P325 (6.7723, -38.4075)
  point P326 (7.4669, -42.3467)
  point P327 (6.7723, -38.4075)
  point P328 (6.7723, -38.4075)
  point P329 (7.2932, -41.3619)
  point P330 (-6.7723, -38.4075)
  point P331 (6.7723, -38.4075)
  point P332 (21, -36.3731)
  point P333 (21.5, -37.2391)
  point P334 (7.4669, -42.3467)
  point P335 (20.944, -31.3236)
  point P336 (19.5, -33.775)
  point P337 (6.7723, -38.4075)
  point P338 (6.7723, -38.4075)
  point P339 (7.2932, -41.3619)
  point P340 (20.3434, -30.6413)
  point P341 (7.2932, -41.3619)
  point P342 (7.4669, -42.3467)
  point P343 (8.9676, -36.5978)
  point P344 (19.5, -33.775)
  point P345 (21.5, -37.2391)
  point P346 (19.5, -33.775)
  point P347 (19.5, -33.775)
  point P348 (21, -36.3731)
  point P349 (6.7723, -38.4075)
  point P350 (19.5, -33.775)
  point P351 (32.1739, -26.9971)
  point P352 (32.9399, -27.6399)
  point P353 (21.5, -37.2391)
  point P354 (30.3942, -22.2713)
  point P355 (29.8757, -25.0687)
  point P356 (19.5, -33.775)
  point P357 (19.5, -33.775)
  point P358 (21, -36.3731)
  point P359 (29.5965, -21.8356)
  point P360 (21, -36.3731)
  point P361 (21.5, -37.2391)
  point P362 (20.944, -31.3236)
  point P363 (29.8757, -25.0687)
  point P364 (32.9399, -27.6399)
  point P365 (29.8757, -25.0687)
  point P366 (29.8757, -25.0687)
  point P367 (32.1739, -26.9971)
  point P368 (19.5, -33.775)
  point P369 (29.8757, -25.0687)
  point P370 (39.4671, -14.3648)
  point P371 (40.4068, -14.7069)
  point P372 (32.9399, -27.6399)
  point P373 (36.1784, -10.5327)
  point P374 (36.648, -13.3388)
  point P375 (29.8757, -25.0687)
  point P376 (29.8757, -25.0687)
  point P377 (32.1739, -26.9971)
  point P378 (35.2798, -10.3962)
  point P379 (32.1739, -26.9971)
  point P380 (32.9399, -27.6399)
  point P381 (30.3942, -22.2713)
  point P382 (36.648, -13.3388)
  point P383 (40.4068, -14.7069)
  point P384 (36.648, -13.3388)
  point P385 (36.648, -13.3388)
  point P386 (39.4671, -14.3648)
  point P387 (29.8757, -25.0687)
  point P388 (36.648, -13.3388)
  point P389 (42, 0)
  point P390 (43, 0)
  point P391 (40.4068, -14.7069)
  point P392 (37.599, 2.4762)
  point P393 (39, 0)
  point P394 (36.648, -13.3388)
  point P395 (36.648, -13.3388)
  point P396 (39.4671, -14.3648)
  point P397 (36.7079, 2.2972)
  point P398 (39.4671, -14.3648)
  point P399 (40.4068, -14.7069)
  point P400 (36.1784, -10.5327)
  point P401 (39, 0)
  point P402 (43, 0)
  point P403 (39, 0)
  point P404 (39, 0)
  point P405 (42, 0)
  point P406 (36.648, -13.3388)
  point P407 (39, 0)
  point P408 (39.4671, 14.3648)
  point P409 (40.4068, 14.7069)
  point P410 (43, 0)
  point P411 (34.4846, 15.1865)
  point P412 (36.648, 13.3388)
  point P413 (39, 0)
  point P414 (39, 0)
  point P415 (42, 0)
  point P416 (33.7084, 14.7135)
  point P417 (42, 0)
  point P418 (43, 0)
  point P419 (37.599, 2.4762)
  point P420 (36.648, 13.3388)
  point P421 (40.4068, 14.7069)
  point P422 (36.648, 13.3388)
  point P423 (36.648, 13.3388)
  point P424 (39.4671, 14.3648)
  point P425 (39, 0)
  point P426 (36.648, 13.3388)
  point P427 (32.1739, 26.9971)
  point P428 (32.9399, 27.6399)
  point P429 (40.4068, 14.7069)
  point P430 (27.2108, 26.0651)
  point P431 (29.8757, 25.0687)
  point P432 (36.648, 13.3388)
  point P433 (36.648, 13.3388)
  point P434 (39.4671, 14.3648)
  point P435 (26.6432, 25.3551)
  point P436 (39.4671, 14.3648)
  point P437 (40.4068, 14.7069)
  point P438 (34.4846, 15.1865)
  point P439 (29.8757, 25.0687)
  point P440 (32.9399, 27.6399)
  point P441 (29.8757, 25.0687)
  point P442 (29.8757, 25.0687)
  point P443 (32.1739, 26.9971)
  point P444 (36.648, 13.3388)
  point P445 (29.8757, 25.0687)
  point P446 (21, 36.3731)
  point P447 (21.5, 37.2391)
  point P448 (32.9399, 27.6399)
  point P449 (16.655, 33.7998)
  point P450 (19.5, 33.775)
  point P451 (29.8757, 25.0687)
  point P452 (29.8757, 25.0687)
  point P453 (32.1739, 26.9971)
  point P454 (16.3645, 32.9385)
  point P455 (32.1739, 26.9971)
  point P456 (32.9399, 27.6399)
  point P457 (27.2108, 26.0651)
  point P458 (19.5, 33.775)
  point P459 (21.5, 37.2391)
  point P460 (19.5, 33.775)
  point P461 (19.5, 33.775)
  point P462 (21, 36.3731)
  point P463 (29.8757, 25.0687)
  point P464 (19.5, 33.775)
  point P465 (7.2932, 41.3619)
  point P466 (7.4669, 42.3467)
  point P467 (21.5, 37.2391)
  point P468 (4.0904, 37.4578)
  point P469 (6.7723, 38.4075)
  point P470 (19.5, 33.775)
  point P471 (19.5, 33.775)
  point P472 (21, 36.3731)
  point P473 (4.112, 36.5491)
  point P474 (21, 36.3731)
  point P475 (21.5, 37.2391)
  point P476 (16.655, 33.7998)
  point P477 (6.7723, 38.4075)
  point P478 (7.4669, 42.3467)
  point P479 (6.7723, 38.4075)
  point P480 (6.7723, 38.4075)
  point P481 (7.2932, 41.3619)
  point P482 (19.5, 33.775)
  dimension "d3" = 86
  dimension "d4" = 10
  dimension "d5" = 10
  dimension "d6" = 10
  dimension "d12" = 5
  dimension "d29" = 42.9
  dimension "d30" = 4.9996
  dimension "d31" = 1.5
  dimension "d32" = 0.5
  dimension "d33" = 1.5
  dimension "d34" = 0.5
  dimension "d44" = 0.55
  dimension "d45" = 0.5
  dimension "d47" = 360
  dimension "d48" = 98
  constraint coincident L3.start A0.centre
  constraint vertical L4
  constraint coincident L0.start A1
  constraint perpendicular L0 L6
  constraint coincident P468 L6
  constraint coincident P468 P0
  constraint perpendicular L5 L9
  constraint parallel L8 L10
  constraint coincident L9 L5.start
  constraint coincident P478 L3
  constraint coincident L3 L11.end
  constraint coincident P478 P466
  constraint perpendicular L0 L8
  constraint perpendicular L8 L12
  constraint perpendicular L12 L13
  constraint perpendicular L6 L15
  constraint perpendicular L15 L16
  constraint parallel L9 L17
  constraint perpendicular L19 L39
  constraint coincident A5 L39.end
  constraint tangent L14 A22
  constraint tangent L1 A22
  constraint coincident L9 L40.start
  constraint parallel L9 L40
  constraint tangent L41 A23
  constraint tangent L40 A23
  constraint concentric A33 A75
  constraint horizontal L399
  constraint coincident L41.start L399
  measures "d3" diameter of A1
  measures "d4" angle of L3 L4
  measures "d5" angle of L1 L4
  measures "d6" distance of L0.start L0.end
  measures "d12" distance of L0.start L8.end
  measures "d29" distance of L0.end L3.start
  measures "d30" vertical distance of L0.start L8.end
  measures "d31" distance of L8.end L12.end
  measures "d32" distance of L12.end L13.end
  measures "d33" distance of P468 L15.end
  measures "d34" distance of L15.end L16.end
  measures "d44" radius of A22
  measures "d45" radius of A23
  measures "d48" diameter of A75
extrude "Extrude4" add sketch "Sketch1" along normal blind 40 contours L2 L7 L8 L10 L12 L13 L14 L18 A22 L46 | L11 L387 L390 L391 L394 A73 L395 L396 L397 L398 | L51 L54 L55 L58 A25 L59 L60 L61 L62 L67 | L366 L369 L370 L373 A70 L374 L375 L376 L377 L382 | L72 L75 L76 L79 A28 L80 L81 L82 L83 L88 | L345 L348 L349 L352 A67 L353 L354 L355 L356 L361 | L93 L96 L97 L100 A31 L101 L102 L103 L104 L109 | L324 L327 L328 L331 A64 L332 L333 L334 L335 L340 | L114 L117 L118 L121 A34 L122 L123 L124 L125 L130 | L303 L306 L307 L310 A61 L311 L312 L313 L314 L319 | L135 L138 L139 L142 A37 L143 L144 L145 L146 L151 | L282 L285 L286 L289 A58 L290 L291 L292 L293 L298 | L156 L159 L160 L163 A40 L164 L165 L166 L167 L172 | L261 L264 L265 L268 A55 L269 L270 L271 L272 L277 | L177 L180 L181 L184 A43 L185 L186 L187 L188 L193 | L28 L29 L31 L240 L243 L244 L247 A52 L248 L249 L250 L251 L256 | L198 L201 L202 L205 A46 L206 L207 L208 L209 L214 | L219 L222 L223 L226 A49 L227 L228 L229 L230 L235 | A75